Autodesk Fusion 360 part; units mm, degrees
note: some values were not read from the file. Chosen so that the rebuilt part matches the saved one: which face or edge a step refers to. Set by a fixed rule: which sketch regions a step uses; the direction of a hole.
(part 2 of 4)
sketch "Sketch67" plane through (0, 220, 0) normal (0, 1, 0) x (-1, 0, 0)
  line L0 (25, 0) -> (85, 0)
  line L1 (85, 0) -> (85, 30)
  line L2 (80, 25) -> (30, 25)
  line L3 (25, 30) -> (25, 0)
  line L4 (35, 26.3798) -> (35, 15.6202)
  line L5 (30.25, 21) -> (39.75, 21)
  line L6 (39.75, 21) -> (39.75, 17.5)
  line L7 (39.75, 17.5) -> (30.25, 17.5)
  line L8 (30.25, 17.5) -> (30.25, 21)
  line L9 (79.75, 21) -> (70.25, 21)
  line L10 (70.25, 21) -> (70.25, 17.5)
  line L11 (70.25, 17.5) -> (79.75, 17.5)
  line L12 (79.75, 17.5) -> (79.75, 21)
  line L13 (75, 25) -> (75, 17)
  line L14 (25, 25) -> (85, 25)
  line L15 (85, 30) -> (80, 30)
  line L16 (80, 30) -> (80, 25)
  line L17 (30, 25) -> (30, 30)
  line L18 (30, 30) -> (25, 30)
  dimension "d520" = 9.5
  dimension "d521" = 3.5
  dimension "d522" = 4
  dimension "d523" = 10
  dimension "d524" = 9.5
  dimension "d525" = 3.5
  dimension "d526" = 10
  dimension "d527" = 4
  constraint vertical L4
  constraint horizontal L5
  constraint vertical L6
  constraint horizontal L7
  constraint vertical L8
  constraint midpoint L4 L5
  constraint horizontal L9
  constraint vertical L10
  constraint horizontal L11
  constraint vertical L12
  constraint coincident L2 L13.start
  constraint perpendicular L2 L13
  constraint midpoint L9 L13
  measures "d520" distance of L5.start L5.end
  measures "d521" distance of L5.start L7.end
  measures "d522" distance of L2 L5
  measures "d523" distance of L3 L4
  measures "d524" distance of L9.start L9.end
  measures "d525" distance of L9.start L11.end
  measures "d526" distance of L1 L13
  measures "d527" distance of L9 L14
extrude "Extrude94" cut sketch "Sketch67" against normal blind 8 contours L4 L5 L6 L7 | L4 L5 L7 L8 | L9 L11 L12 L13 | L9 L10 L11 L13 bodies 3
sketch "Sketch68" plane through (0, 0, 25) normal (0, 0, 1) x (-1, 0, 0)
  line L0 (-25, -115) -> (-25, -75)
  line L1 (-25, -75) -> (-85, -75)
  line L2 (-85, -75) -> (-85, -115)
  line L3 (-85, -115) -> (-25, -115)
  line L4 (-85, -75) -> (-65, -75)
  line L5 (-65, -75) -> (-65, -115)
  line L6 (-65, -115) -> (-85, -115)
  line L7 (-85, -115) -> (-85, -75)
  constraint horizontal L4
  constraint vertical L5
  constraint horizontal L6
  constraint vertical L7
  constraint coincident L3 L5.end
  constraint coincident L1.end L2.start
sketch "Sketch70" plane through (85, 0, 0) normal (1, 0, 0) x (0, 1, 0)
  line L0 (115, 25) -> (115, 60)
  line L1 (115, 60) -> (75, 60)
  line L2 (75, 60) -> (75, 25)
  line L3 (75, 10) -> (115, 10)
  line L4 (75, 10) -> (75, 20)
  line L5 (115, 20) -> (75, 20)
  line L6 (115, 20) -> (115, 10)
  line L7 (75, 60) -> (115, 60)
  line L8 (115, 60) -> (115, 57)
  line L9 (115, 57) -> (75, 57)
  line L10 (75, 57) -> (75, 60)
  line L11 (75, 25) -> (115, 25)
  dimension "d537" = 40
  constraint coincident L0 L3.end
  constraint perpendicular L0 L3
  constraint coincident L2 L4.end
  constraint coincident L0 L5.start
  constraint perpendicular L4 L5
  constraint horizontal L7
  constraint vertical L8
  constraint horizontal L9
  constraint vertical L10
  constraint coincident L0 L8.end
  constraint coincident L1.end L2.start
  measures "d537" distance of L1 L5
sketch "Sketch71" plane through (0, 0, 57) normal (0, 0, -1) x (1, 0, 0)
  line L0 (85, -115) -> (93, -115)
  line L1 (93, -115) -> (93, -75)
  line L2 (93, -75) -> (85, -75)
  circle A0 centre (90.65, -110.5) radius 1.5
  line L3 (85, -115) -> (85, -75)
  circle A1 centre (90.65, -79.5) radius 1.5
  line L4 (85, -75) -> (85, -115)
  dimension "d543" = 3
  dimension "d544" = 5.65
  dimension "d545" = 3
  dimension "d546" = 5.65
  dimension "d547" = 31
  dimension "d548" = 4.5
  measures "d543" diameter of A0
  measures "d544" distance of A0.centre L3
  measures "d545" diameter of A1
  measures "d546" distance of L3 A1.centre
  measures "d547" distance of A0.centre A1.centre
  measures "d548" distance of L2 A1.centre
sketch "Sketch72" plane through (0, 0, 20) normal (0, 0, 1) x (-1, 0, 0)
  line L0 (-85, -75) -> (-95, -75)
  line L1 (-95, -75) -> (-95, -115)
  line L2 (-95, -115) -> (-85, -115)
  circle A0 centre (-106.15, -95) radius 9.5
  line L3 (-85, -75) -> (-85, -115)
  line L4 (-85, -115) -> (-85, -75)
  dimension "d552" = 19
  dimension "d553" = 21.15
  dimension "d554" = 20
  measures "d552" diameter of A0
  measures "d553" distance of A0.centre L3
  measures "d554" distance of L2 A0.centre
sketch "Sketch73" plane through (0, 115, 0) normal (0, 1, 0) x (-1, 0, 0)
  line L0 (-85, 60) -> (-93, 60)
  line L1 (-93, 60) -> (-93, 57)
  line L2 (-93, 57) -> (-85, 57)
  circle A0 centre (-55, 45) radius 10
  line L3 (-85, 57) -> (-85, 60)
sketch "Sketch74" plane through (0, 0, 90) normal (0, 0, 1) x (-1, 0, 0)
  circle A0 centre (-106.15, -95) radius 9.5
  circle A1 centre (-106.15, -95) radius 4
  dimension "d563" = 8
  constraint concentric A0 A1
  measures "d563" diameter of A1
sketch "Sketch76" plane through (0, 0, 60) normal (0, 0, 1) x (-1, 0, 0)
  circle A0 centre (-90.65, -110.5) radius 1.5
  circle A1 centre (-90.65, -79.5) radius 1.5
  line L0 (-93, -115) -> (-85, -115)
  line L1 (-85, -75) -> (-93, -75)
  line L2 (-93, -75) -> (-93, -115)
  line L3 (-80, -90) -> (-70, -90)
  line L4 (-70, -90) -> (-70, -100)
  line L5 (-70, -100) -> (-80, -100)
  line L6 (-80, -100) -> (-80, -90)
  line L7 (-85, -115) -> (-85, -75)
  dimension "d566" = 10
  dimension "d567" = 10
  constraint horizontal L3
  constraint vertical L4
  constraint horizontal L5
  constraint vertical L6
  measures "d566" distance of L3.start L3.end
  measures "d567" distance of L3.start L5.end
sketch "Sketch77" plane through (0, 0, 0) normal (0, 0, 1) x (1, 0, 0)
  line L0 (145, 120) -> (60, 120)
  line L1 (60, 120) -> (60, 150)
  line L2 (60, 150) -> (145, 150)
  line L3 (145, 150) -> (145, 120)
  dimension "d669" = 85
  constraint horizontal L0
  constraint vertical L1
  constraint horizontal L2
  constraint vertical L3
  measures "d669" distance of L1.end L2.end
sketch "Sketch78" plane through (0, 0, 10) normal (0, 0, 1) x (-1, 0, 0)
  line L0 (-145, -150) -> (-60, -150)
  line L1 (-60, -150) -> (-60, -120)
  line L2 (-60, -120) -> (-145, -120)
  line L3 (-145, -120) -> (-145, -150)
  circle A0 centre (-103.65, -135) radius 8.5
  line L4 (-77.5, -130) -> (-67.5, -130)
  line L5 (-67.5, -130) -> (-67.5, -140)
  line L6 (-67.5, -140) -> (-77.5, -140)
  line L7 (-77.5, -140) -> (-77.5, -130)
  circle A1 centre (-67.5, -130) radius 1.5
  circle A2 centre (-67.5, -140) radius 1.5
  circle A3 centre (-77.5, -140) radius 1.5
  circle A4 centre (-77.5, -130) radius 1.5
  circle A5 centre (-72.5, -135) radius 2.5
  line L8 (-139.8, -130) -> (-129.8, -130)
  line L9 (-129.8, -130) -> (-129.8, -140)
  line L10 (-129.8, -140) -> (-139.8, -140)
  line L11 (-139.8, -140) -> (-139.8, -130)
  line L12 (-145, -150) -> (-145, -120)
  line L13 (-60, -150) -> (-145, -150)
  circle A6 centre (-129.8, -130) radius 1.5
  circle A7 centre (-129.8, -140) radius 1.5
  circle A8 centre (-139.8, -130) radius 1.5
  circle A9 centre (-139.8, -140) radius 1.5
  circle A10 centre (-134.8, -135) radius 2.5
  dimension "d572" = 17
  dimension "d573" = 26.15
  dimension "d574" = 7.5
  dimension "d582" = 5
  dimension "d583" = 5
  dimension "d584" = 5
  dimension "d670" = 10
  dimension "d671" = 10
  dimension "d674" = 3
  dimension "d675" = 3
  dimension "d676" = 3
  dimension "d677" = 3
  dimension "d678" = 5
  dimension "d679" = 26.15
  dimension "d680" = 10
  dimension "d681" = 5
  constraint horizontal L4
  constraint vertical L5
  constraint horizontal L6
  constraint vertical L7
  constraint coincident L4.end L5.start
  constraint coincident L5.end L6.start
  constraint coincident L6.end L7.start
  constraint coincident L4.start L7.end
  constraint horizontal L8
  constraint vertical L9
  constraint horizontal L10
  constraint vertical L11
  constraint coincident L8.end L9.start
  constraint coincident L9.end L10.start
  constraint coincident L8.start L11.end
  constraint coincident L10.end L11.start
  measures "d572" diameter of A0
  measures "d573" distance of A0.centre L7
  measures "d574" distance of L1 L5
  measures "d582" distance of L4 A5.centre
  measures "d583" distance of L7 A5.centre
  measures "d584" diameter of A5
  measures "d670" distance of L8.start L8.end
  measures "d671" distance of L8.start L10.end
  measures "d674" diameter of A6
  measures "d675" diameter of A7
  measures "d676" diameter of A8
  measures "d677" diameter of A9
  measures "d678" diameter of A10
  measures "d679" distance of A0.centre L9
  measures "d680" distance of L5.end L6.end
  measures "d681" distance of L9 A10.centre
sketch "Sketch79" plane through (0, 0, 140) normal (0, 0, 1) x (-1, 0, 0)
  line L0 (-80, -100) -> (-70, -100)
  line L1 (-70, -100) -> (-70, -90)
  line L2 (-70, -90) -> (-80, -90)
  line L3 (-80, -90) -> (-80, -100)
  circle A0 centre (-75, -95) radius 2.5
  dimension "d587" = 5
  measures "d587" diameter of A0
sketch "Sketch80" plane through (0, 0, 0) normal (0, 0, 1) x (1, 0, 0)
  line L0 (120, 160) -> (25, 160)
  line L1 (25, 160) -> (25, 190)
  line L2 (25, 190) -> (120, 190)
  line L3 (120, 190) -> (120, 160)
  dimension "d593" = 95
  dimension "d594" = 30
  constraint horizontal L0
  constraint vertical L1
  constraint horizontal L2
  constraint vertical L3
  measures "d593" distance of L0.start L0.end
  measures "d594" distance of L0.start L2.end
sketch "Sketch81" plane through (0, 0, 90) normal (0, 0, 1) x (-1, 0, 0)
  circle A0 centre (-90.65, -110.5) radius 1.5
  circle A1 centre (-90.65, -79.5) radius 1.5
  line L0 (-93, -115) -> (-85, -115)
  line L1 (-85, -75) -> (-93, -75)
  line L2 (-93, -75) -> (-93, -115)
  line L3 (-93, -105) -> (-85, -105)
  line L4 (-85, -105) -> (-85, -115)
  line L5 (-85, -115) -> (-93, -115)
  line L6 (-93, -115) -> (-93, -105)
  line L7 (-93, -75) -> (-85, -75)
  line L8 (-85, -75) -> (-85, -85)
  line L9 (-85, -85) -> (-93, -85)
  line L10 (-93, -85) -> (-93, -75)
  line L11 (-85, -115) -> (-85, -75)
  constraint horizontal L3
  constraint vertical L4
  constraint horizontal L5
  constraint vertical L6
  constraint coincident L0 L4.end
  constraint coincident L2 L3.start
  constraint horizontal L7
  constraint vertical L8
  constraint horizontal L9
  constraint vertical L10
  constraint coincident L1.end L2.start
extrude "Extrude108" cut sketch "Sketch81" against normal blind 23 contours L0 L2 L3 L4 L5 L6 L11 | L1 L2 L7 L8 L9 L10 L11
sketch "Sketch82" plane through (0, 0, 15) normal (0, 0, 1) x (-1, 0, 0)
  line L0 (-120, -190) -> (-25, -190)
  line L1 (-25, -190) -> (-25, -160)
  line L2 (-25, -160) -> (-120, -160)
  line L3 (-120, -160) -> (-120, -190)
  circle A0 centre (-103.65, -175) radius 7.5
  line L4 (-77.5, -170) -> (-67.5, -170)
  line L5 (-67.5, -170) -> (-67.5, -180)
  line L6 (-67.5, -180) -> (-77.5, -180)
  line L7 (-77.5, -180) -> (-77.5, -170)
  circle A1 centre (-67.5, -170) radius 1.5
  circle A2 centre (-67.5, -180) radius 1.5
  circle A3 centre (-77.5, -180) radius 1.5
  circle A4 centre (-77.5, -170) radius 1.5
  line L8 (-57.5, -160) -> (-57.5, -190)
  line L9 (-47.5, -160) -> (-47.5, -190)
  dimension "d603" = 15
  dimension "d604" = 26.15
  dimension "d605" = 16.35
  dimension "d606" = 10
  dimension "d607" = 10
  constraint horizontal L4
  constraint vertical L5
  constraint horizontal L6
  constraint vertical L7
  constraint coincident L4.end L5.start
  constraint coincident L5.end L6.start
  constraint coincident L6.end L7.start
  constraint coincident L4.start L7.end
  constraint coincident L2 L8.start
  constraint coincident L0 L8.end
  constraint perpendicular L0 L8
  constraint coincident L2 L9.start
  constraint coincident L0 L9.end
  constraint perpendicular L0 L9
  measures "d603" diameter of A0
  measures "d604" distance of A0.centre L7
  measures "d605" distance of L3 A0.centre
  measures "d606" distance of L5 L8
  measures "d607" distance of L8 L9
sketch "Sketch89" plane through (0, 190, 0) normal (0, 1, 0) x (-1, 0, 0)
  line L0 (-47.5, 15) -> (-47.5, 65)
  line L1 (-47.5, 65) -> (-57.5, 65)
  line L2 (-57.5, 65) -> (-57.5, 15)
  circle A0 centre (-47.5, 55) radius 10
  line L3 (-57.5, 15) -> (-47.5, 15)
  dimension "d623" = 20
  constraint tangent L1 A0
  constraint tangent L2 A0
  measures "d623" diameter of A0
sketch "Sketch90" plane through (0, 0, 65) normal (0, 0, 1) x (-1, 0, 0)
  line L0 (-57.5, -160) -> (-57.5, -190)
  line L1 (-57.5, -190) -> (-47.5, -190)
  line L2 (-47.5, -190) -> (-47.5, -160)
  line L3 (-47.5, -160) -> (-57.5, -160)
  line L4 (-47.5, -190) -> (-47.5, -198)
  line L5 (-47.5, -160) -> (-40, -160)
  line L6 (-40, -160) -> (-40, -198)
  line L7 (-40, -198) -> (-47.5, -198)
  line L8 (-47.5, -198) -> (-47.5, -160)
  line L9 (-40, -198) -> (-150, -198)
  line L10 (-150, -198) -> (-150, -228)
  line L11 (-150, -228) -> (-40, -228)
  line L12 (-40, -228) -> (-40, -198)
  circle A0 centre (-47.5, -198) radius 1.5
  circle A1 centre (-68, -223) radius 1.5
  circle A2 centre (-140, -223) radius 1.5
  line L13 (-150, -228) -> (-40, -228)
  point P0 (-47.5, -190)
  dimension "d643" = 8
  dimension "d644" = 110
  dimension "d645" = 30
  dimension "d652" = 3
  dimension "d655" = 3
  dimension "d656" = 3
  dimension "d657" = 25
  dimension "d658" = 25
  dimension "d659" = 72
  dimension "d660" = 28
  dimension "d733" = 8
  constraint coincident P0 L1.end
  constraint perpendicular L1 L4
  constraint horizontal L5
  constraint vertical L6
  constraint horizontal L7
  constraint vertical L8
  constraint coincident L2.end L3.start
  constraint horizontal L9
  constraint vertical L10
  constraint horizontal L11
  constraint vertical L12
  constraint coincident L4.end L7.end
  constraint horizontal L13
  measures "d643" distance of P0 L4.end
  measures "d644" distance of L6.end L9.end
  measures "d645" distance of L6.end L11.end
  measures "d652" diameter of A0
  measures "d655" diameter of A1
  measures "d656" diameter of A2
  measures "d657" distance of L9 A1.centre
  measures "d658" distance of L9 A2.centre
  measures "d659" distance of A1.centre A2.centre
  measures "d660" distance of L12 A1.centre
  measures "d733" distance of L9 P0
sketch "Sketch92" plane through (0, 0, 0) normal (0, 0, 1) x (1, 0, 0)
sketch "Sketch93" plane through (0, 0, 0) normal (0, 0, 1) x (1, 0, 0)
  line L0 (160.9039, 76.8073) -> (132.9039, 76.8073)
  line L1 (132.9039, 76.8073) -> (132.9039, 116.8073)
  line L2 (132.9039, 116.8073) -> (160.9039, 116.8073)
  line L3 (160.9039, 116.8073) -> (160.9039, 76.8073)
  line L4 (160.9039, 76.8073) -> (152.9039, 76.8073)
  line L5 (152.9039, 76.8073) -> (152.9039, 86.8073)
  line L6 (152.9039, 86.8073) -> (160.9039, 86.8073)
  line L7 (160.9039, 86.8073) -> (160.9039, 76.8073)
  line L8 (160.9039, 116.8073) -> (152.9039, 116.8073)
  line L9 (152.9039, 116.8073) -> (152.9039, 106.8073)
  line L10 (152.9039, 106.8073) -> (160.9039, 106.8073)
  line L11 (160.9039, 106.8073) -> (160.9039, 116.8073)
  line L12 (147.9039, 91.8073) -> (137.9039, 91.8073)
  line L13 (137.9039, 91.8073) -> (137.9039, 101.8073)
  line L14 (137.9039, 101.8073) -> (147.9039, 101.8073)
  line L15 (147.9039, 101.8073) -> (147.9039, 91.8073)
  circle A0 centre (158.5539, 112.3073) radius 1.5
  circle A1 centre (158.5539, 81.3073) radius 1.5
  line L16 (152.9039, 106.8073) -> (152.9039, 86.8073)
  dimension "d686" = 28
  dimension "d687" = 40
  dimension "d688" = 8
  dimension "d689" = 10
  dimension "d690" = 8
  dimension "d691" = 10
  dimension "d692" = 10
  dimension "d693" = 10
  dimension "d694" = 15
  dimension "d695" = 5
  dimension "d700" = 3
  dimension "d701" = 3
  dimension "d702" = 2.35
  dimension "d703" = 4.5
  dimension "d704" = 2.35
  dimension "d705" = 4.5
  constraint horizontal L0
  constraint vertical L1
  constraint horizontal L2
  constraint vertical L3
  constraint horizontal L4
  constraint vertical L5
  constraint horizontal L6
  constraint vertical L7
  constraint horizontal L8
  constraint vertical L9
  constraint horizontal L10
  constraint vertical L11
  constraint horizontal L12
  constraint vertical L13
  constraint horizontal L14
  constraint vertical L15
  measures "d686" distance of L0.start L0.end
  measures "d687" distance of L0.start L2.end
  measures "d688" distance of L0.start L4.end
  measures "d689" distance of L0.start L6.end
  measures "d690" distance of L2.end L8.end
  measures "d691" distance of L2.end L10.end
  measures "d692" distance of L12.start L12.end
  measures "d693" distance of L12.start L14.end
  measures "d694" distance of L2 L14
  measures "d695" distance of L1 L13
  measures "d700" diameter of A0
  measures "d701" diameter of A1
  measures "d702" distance of L11 A0.centre
  measures "d703" distance of L8 A0.centre
  measures "d704" distance of L3 A1.centre
  measures "d705" distance of L4 A1.centre
sketch "Sketch94" plane through (152.9039, 0, 0) normal (1, 0, 0) x (0, 1, 0)
  line L0 (76.8073, 0) -> (76.8073, -47)
  line L1 (76.8073, -47) -> (116.8073, -47)
  line L2 (116.8073, -47) -> (116.8073, 0)
  line L3 (76.8073, -47) -> (116.8073, -47)
  line L4 (116.8073, -47) -> (116.8073, -38)
  line L5 (116.8073, -38) -> (76.8073, -38)
  line L6 (76.8073, -38) -> (76.8073, -47)
  line L7 (116.8073, 0) -> (76.8073, 0)
  dimension "d712" = 9
  constraint horizontal L3
  constraint vertical L4
  constraint horizontal L5
  constraint vertical L6
  constraint coincident L2 L4.end
  constraint coincident L0.end L1.start
  measures "d712" distance of L0.end L5.end
sketch "Sketch95" plane through (0, 0, 15) normal (0, 0, 1) x (-1, 0, 0)
  line L0 (-120, -160) -> (-147.5, -160)
  line L1 (-147.5, -160) -> (-147.5, -190)
  line L2 (-147.5, -190) -> (-120, -190)
  line L3 (-129.8, -180) -> (-139.8, -180)
  line L4 (-139.8, -180) -> (-139.8, -170)
  line L5 (-139.8, -170) -> (-129.8, -170)
  line L6 (-129.8, -170) -> (-129.8, -180)
  circle A0 centre (-139.8, -180) radius 1.5
  circle A1 centre (-139.8, -170) radius 1.5
  circle A2 centre (-129.8, -170) radius 1.5
  circle A3 centre (-129.8, -180) radius 1.5
  line L7 (-120, -190) -> (-120, -160)
  point P0 (-103.65, -175)
  dimension "d717" = 10
  dimension "d718" = 10
  dimension "d719" = 26.15
  dimension "d720" = 10
  dimension "d721" = 3
  dimension "d722" = 3
  dimension "d723" = 3
  dimension "d724" = 3
  constraint horizontal L3
  constraint vertical L4
  constraint horizontal L5
  constraint vertical L6
  constraint coincident L3.end L4.start
  constraint coincident L4.end L5.start
  constraint coincident L5.end L6.start
  constraint coincident L3.start L6.end
  measures "d717" distance of L3.start L3.end
  measures "d718" distance of L3.start L5.end
  measures "d719" distance of L6 P0
  measures "d720" distance of L0 L5
  measures "d721" diameter of A0
  measures "d722" diameter of A1
  measures "d723" diameter of A2
  measures "d724" diameter of A3
sketch "Sketch96" plane through (0, 0, 83) normal (0, 0, 1) x (-1, 0, 0)
  line L0 (-147.9039, -101.8073) -> (-137.9039, -101.8073)
  line L1 (-137.9039, -101.8073) -> (-137.9039, -91.8073)
  line L2 (-137.9039, -91.8073) -> (-147.9039, -91.8073)
  line L3 (-147.9039, -91.8073) -> (-147.9039, -101.8073)
  circle A0 centre (-142.9039, -96.8073) radius 2.5
  dimension "d727" = 5
  measures "d727" diameter of A0
sketch "Sketch97" plane through (0, 0, 15) normal (0, 0, 1) x (-1, 0, 0)
  line L0 (-149.8, -190) -> (-149.8, -160)
  line L1 (-139.8, -180) -> (-139.8, -170)
  line L2 (-147.5, -190) -> (-149.8, -190)
  line L3 (-149.8, -160) -> (-147.5, -160)
  line L4 (-149.8, -190) -> (-159.8, -190)
  line L5 (-159.8, -190) -> (-159.8, -160)
  line L6 (-159.8, -160) -> (-149.8, -160)
  line L7 (-149.8, -160) -> (-149.8, -190)
  line L8 (-147.5, -190) -> (-147.5, -160)
  dimension "d734" = 10
  dimension "d735" = 10
  constraint vertical L0
  constraint perpendicular L0 L2
  constraint perpendicular L0 L3
  constraint horizontal L4
  constraint vertical L5
  constraint horizontal L6
  constraint vertical L7
  constraint perpendicular L3 L8
  measures "d734" distance of L0 L1
  measures "d735" distance of L0.start L4.end
sketch "Sketch98" plane through (0, 0, 15) normal (0, 0, 1) x (-1, 0, 0)
sketch "Sketch99" plane through (0, 190, 0) normal (0, 1, 0) x (-1, 0, 0)
  line L0 (-149.8, 15) -> (-149.8, 65)
  line L1 (-149.8, 65) -> (-159.8, 65)
  line L2 (-159.8, 65) -> (-159.8, 15)
  circle A0 centre (-159.8, 55) radius 10
  line L3 (-159.8, 55) -> (-169.8, 55)
  line L4 (-159.8, 55) -> (-167.3, 55)
  line L5 (-167.3, 55) -> (-167.3, 65)
  line L6 (-167.3, 65) -> (-159.8, 65)
  line L7 (-159.8, 65) -> (-159.8, 55)
  line L8 (-159.8, 15) -> (-149.8, 15)
  dimension "d740" = 20
  dimension "d741" = 7.5
  constraint coincident L2 A0.centre
  constraint tangent L1 A0
  constraint coincident A0.centre L3.start
  constraint coincident A0 L3.end
  constraint perpendicular L2 L3
  constraint horizontal L4
  constraint vertical L5
  constraint horizontal L6
  constraint vertical L7
  measures "d740" diameter of A0
  measures "d741" distance of A0.centre L4.end
sketch "Sketch100" plane through (0, 0, 0) normal (0, 0, 1) x (1, 0, 0)
  line L0 (50, 0) -> (110, 0)
  line L1 (110, 0) -> (110, -45)
  line L2 (110, -45) -> (50, -45)
  line L3 (50, -45) -> (50, 0)
  dimension "d752" = 60
  dimension "d753" = 45
  constraint horizontal L0
  constraint vertical L1
  constraint horizontal L2
  constraint vertical L3
  measures "d752" distance of L0.start L0.end
  measures "d753" distance of L0.start L2.end
extrude "Extrude139" add sketch "Sketch100" along normal blind 30 separate body makes body 5
sketch "Sketch101" plane through (0, -45, 0) normal (0, -1, 0) x (1, 0, 0)
  line L0 (50, 0) -> (110, 0)
  line L1 (110, 0) -> (110, 30)
  line L2 (110, 30) -> (50, 30)
  line L3 (50, 30) -> (50, 0)
  line L4 (55, 5) -> (60, 5)
  line L5 (60, 5) -> (60, 0)
  line L6 (60, 0) -> (55, 0)
  line L7 (55, 0) -> (55, 5)
  line L8 (100, 5) -> (105, 5)
  line L9 (105, 5) -> (105, 0)
  line L10 (105, 0) -> (100, 0)
  line L11 (100, 0) -> (100, 5)
  line L12 (55, 5) -> (54, 5)
  line L13 (54, 5) -> (55, 0)
  line L14 (60, 5) -> (61, 5)
  line L15 (60, 0) -> (61, 5)
  line L16 (100, 5) -> (99, 5)
  line L17 (99, 5) -> (100, 0)
  line L18 (105, 5) -> (106, 5)
  line L19 (106, 5) -> (105, 0)
  line L20 (80, 0) -> (80, 12.75)
  circle A0 centre (80, 12.75) radius 7.5
  circle A1 centre (54, 5) radius 1
  circle A2 centre (61, 5) radius 1
  circle A3 centre (60, 0) radius 1
  circle A4 centre (55, 0) radius 1
  circle A5 centre (99, 5) radius 1
  circle A6 centre (106, 5) radius 1
  circle A7 centre (105, 0) radius 1
  circle A8 centre (100, 0) radius 1
  dimension "d756" = 1
  dimension "d757" = 1
  dimension "d758" = 1
  dimension "d759" = 1
  dimension "d760" = 12.75
  dimension "d761" = 15
  dimension "d762" = 2
  dimension "d763" = 2
  dimension "d764" = 2
  dimension "d765" = 2
  dimension "d766" = 2
  dimension "d767" = 2
  dimension "d768" = 2
  dimension "d769" = 2
  constraint horizontal L4
  constraint vertical L5
  constraint horizontal L6
  constraint vertical L7
  constraint coincident L0 L5.end
  constraint horizontal L8
  constraint vertical L9
  constraint horizontal L10
  constraint vertical L11
  constraint coincident L0 L9.end
  constraint perpendicular L7 L12
  constraint perpendicular L7 L14
  constraint perpendicular L11 L16
  constraint perpendicular L9 L18
  constraint midpoint L0 L20.start
  constraint perpendicular L0 L20
  constraint coincident L20.end A0.centre
  constraint coincident L12.end L13.start
  constraint coincident L14.end L15.end
  constraint coincident L5.end L6.start
  constraint coincident L6.end L7.start
  constraint coincident L16.end L17.start
  constraint coincident L18.end L19.start
  constraint coincident L9.end L10.start
  constraint coincident L10.end L11.start
  measures "d756" distance of L4.start L12.end
  measures "d757" distance of L4.end L14.end
  measures "d758" distance of L8.start L16.end
  measures "d759" distance of L8.end L18.end
  measures "d760" distance of L20.start L20.end
  measures "d761" diameter of A0
  measures "d762" diameter of A1
  measures "d763" diameter of A2
  measures "d764" diameter of A3
  measures "d765" diameter of A4
  measures "d766" diameter of A5
  measures "d767" diameter of A6
  measures "d768" diameter of A7
  measures "d769" diameter of A8
extrude "Extrude140" cut sketch "Sketch101" against normal blind 45 contours L0 L6 L7 A4 | L7 L13 A4 | L0 L13 A4 | L0 L4 L5 L6 L7 A3 A4 | L7 L13 A1 A4 | L0 L5 L6 A3 | L12 L13 A1 | L12 L13 A1 | L0 L15 A3 | L5 L15 A3 | L5 L15 A2 A3 | L14 L15 A2 | L14 L15 A2 | L0 L17 A8 | L0 L10 L11 A8 | L11 L17 A8 | L11 L17 A5 A8 | L0 L8 L9 L10 L11 A7 A8 | L0 L19 A7 | L16 L17 A5 | L16 L17 A5 | L0 L9 L10 A7 | L9 L19 A7 | L9 L19 A6 A7 | L18 L19 A6 | L18 L19 A6 bodies 5
hole "Hole30" at (80, -45, 12.75) direction (0, 1, 0) diameter 13.9 depth 15 tip angle 180 countersink diameter 15 countersink angle 30 bodies 5
sketch "Sketch102" plane through (0, 0, 0) normal (0, 1, 0) x (-1, 0, 0)
  arc A0 (-60.1961, 0.9806) -> (-61, 0) centre (-60, 0) ccw
  line L0 (-60.1961, 0.9806) -> (-60.8039, 4.0194)
  arc A1 (-60, 5) -> (-60.8039, 4.0194) centre (-61, 5) ccw
  line L1 (-60, 5) -> (-55, 5)
  arc A2 (-54.1961, 4.0194) -> (-55, 5) centre (-54, 5) ccw
  line L2 (-54.1961, 4.0194) -> (-54.8039, 0.9806)
  arc A3 (-54, 0) -> (-54.8039, 0.9806) centre (-55, 0) ccw
  line L3 (-54, 0) -> (-50, 0)
  line L4 (-50, 0) -> (-50, 30)
  line L5 (-50, 30) -> (-110, 30)
  line L6 (-110, 30) -> (-110, 0)
  line L7 (-110, 0) -> (-106, 0)
  arc A4 (-105.1961, 0.9806) -> (-106, 0) centre (-105, 0) ccw
  line L8 (-105.1961, 0.9806) -> (-105.8039, 4.0194)
  arc A5 (-105, 5) -> (-105.8039, 4.0194) centre (-106, 5) ccw
  line L9 (-105, 5) -> (-100, 5)
  arc A6 (-99.1961, 4.0194) -> (-100, 5) centre (-99, 5) ccw
  line L10 (-99.1961, 4.0194) -> (-99.8039, 0.9806)
  arc A7 (-99, 0) -> (-99.8039, 0.9806) centre (-100, 0) ccw
  line L11 (-99, 0) -> (-61, 0)
  line L12 (-80, 0) -> (-80, 12.75)
  circle A8 centre (-80, 12.75) radius 11.5
  dimension "d777" = 12.75
  dimension "d778" = 23
  constraint midpoint L11 L12.start
  constraint perpendicular L11 L12
  constraint coincident L12.end A8.centre
  measures "d777" distance of L12.start L12.end
  measures "d778" diameter of A8
hole "Hole31" at (80, 0, 12.75) direction (0, -1, 0) diameter 21 depth 30 tip angle 180 counterbore diameter 23 counterbore depth 3 bodies 5
sketch "Sketch103" plane through (0, 0, 30) normal (0, 0, 1) x (-1, 0, 0)
  line L0 (-50, 45) -> (-110, 45)
  line L1 (-110, 45) -> (-110, 0)
  line L2 (-110, 0) -> (-50, 0)
  line L3 (-50, 0) -> (-50, 45)
  line L4 (-90, 0) -> (-110, 0)
  line L5 (-110, 0) -> (-110, 45)
  line L6 (-110, 45) -> (-90, 45)
  line L7 (-90, 45) -> (-90, 0)
  constraint horizontal L4
  constraint vertical L5
  constraint horizontal L6
  constraint vertical L7
  constraint coincident L0.end L1.start
  constraint coincident L2 L4.start
extrude "Extrude141" add sketch "Sketch103" along normal blind 60 contours L0 L1 L2 L4 L5 L6 L7 bodies 5
sketch "Sketch104" plane through (0, -45, 0) normal (0, -1, 0) x (1, 0, 0)
  circle A0 centre (80, 12.75) radius 7.5
  arc A1 (61, 0) -> (60.1961, 0.9806) centre (60, 0) ccw
  line L0 (61, 0) -> (99, 0)
  arc A2 (99.8039, 0.9806) -> (99, 0) centre (100, 0) ccw
  line L1 (99.8039, 0.9806) -> (99.1961, 4.0194)
  arc A3 (100, 5) -> (99.1961, 4.0194) centre (99, 5) ccw
  line L2 (100, 5) -> (105, 5)
  arc A4 (105.8039, 4.0194) -> (105, 5) centre (106, 5) ccw
  line L3 (105.8039, 4.0194) -> (105.1961, 0.9806)
  arc A5 (106, 0) -> (105.1961, 0.9806) centre (105, 0) ccw
  line L4 (106, 0) -> (110, 0)
  line L5 (110, 0) -> (110, 90)
  line L6 (110, 90) -> (90, 90)
  line L7 (90, 90) -> (90, 30)
  line L8 (90, 30) -> (50, 30)
  line L9 (50, 30) -> (50, 0)
  line L10 (50, 0) -> (54, 0)
  arc A6 (54.8039, 0.9806) -> (54, 0) centre (55, 0) ccw
  line L11 (54.8039, 0.9806) -> (54.1961, 4.0194)
  arc A7 (55, 5) -> (54.1961, 4.0194) centre (54, 5) ccw
  line L12 (55, 5) -> (60, 5)
  arc A8 (60.8039, 4.0194) -> (60, 5) centre (61, 5) ccw
  line L13 (60.8039, 4.0194) -> (60.1961, 0.9806)
  circle A9 centre (80, 40) radius 10
  constraint tangent L7 A9
extrude "Extrude142" add sketch "Sketch104" against normal blind 45 contours L7 L8 A9 bodies 5
sketch "Sketch105" plane through (110, 0, 0) normal (1, 0, 0) x (0, 1, 0)
  line L0 (-45, 0) -> (0, 0)
  line L1 (0, 0) -> (0, 90)
  line L2 (0, 90) -> (-45, 90)
  line L3 (-45, 90) -> (-45, 0)
  line L4 (-45, 90) -> (0, 90)
  line L5 (0, 90) -> (0, 57)
  line L6 (0, 57) -> (-45, 57)
  line L7 (-45, 57) -> (-45, 90)
  line L8 (-45, 90) -> (-32.5, 90)
  line L9 (-32.5, 90) -> (-32.5, 57)
  line L10 (-32.5, 57) -> (-45, 57)
  line L11 (-45, 57) -> (-45, 90)
  line L12 (0, 90) -> (-12.5, 90)
  line L13 (-12.5, 90) -> (-12.5, 57)
  line L14 (-12.5, 57) -> (0, 57)
  line L15 (0, 57) -> (0, 90)
  line L16 (-45, 57) -> (0, 57)
  line L17 (0, 57) -> (0, 67)
  line L18 (0, 67) -> (-45, 67)
  line L19 (-45, 67) -> (-45, 57)
  line L20 (-45, 0) -> (0, 0)
  line L21 (0, 0) -> (0, 10)
  line L22 (0, 10) -> (-45, 10)
  line L23 (-45, 10) -> (-45, 0)
  line L24 (-45, 10) -> (0, 10)
  line L25 (0, 10) -> (0, 20)
  line L26 (0, 20) -> (-45, 20)
  line L27 (-45, 20) -> (-45, 10)
  dimension "d788" = 33
  dimension "d789" = 12.5
  dimension "d790" = 12.5
  dimension "d791" = 10
  dimension "d792" = 10
  dimension "d793" = 10
  constraint horizontal L4
  constraint vertical L5
  constraint horizontal L6
  constraint vertical L7
  constraint coincident L2.end L3.start
  constraint horizontal L8
  constraint vertical L9
  constraint horizontal L10
  constraint vertical L11
  constraint horizontal L12
  constraint vertical L13
  constraint horizontal L14
  constraint vertical L15
  constraint coincident L1.end L2.start
  constraint horizontal L16
  constraint vertical L17
  constraint horizontal L18
  constraint vertical L19
  constraint coincident L15 L17.end
  constraint horizontal L20
  constraint vertical L21
  constraint horizontal L22
  constraint vertical L23
  constraint coincident L1 L21.end
  constraint coincident L0.start L3.end
  constraint horizontal L24
  constraint vertical L25
  constraint horizontal L26
  constraint vertical L27
  constraint coincident L1 L25.end
  measures "d788" distance of L2.end L6.end
  measures "d789" distance of L2.end L8.end
  measures "d790" distance of L1.end L12.end
  measures "d791" distance of L6.end L18.end
  measures "d792" distance of L0.start L22.end
  measures "d793" distance of L22.end L26.end
extrude "Extrude143" add sketch "Sketch105" along normal blind 8 contours L1 L3 L22 L24 L25 L26 L27 | L3 L6 L7 L9 L10 L11 L16 L18 L19 | L1 L5 L6 L13 L14 L15 L16 L17 L18 | L6 L9 L13 L16 L18 | L2 L4 L9 L13 L18 bodies 5
sketch "Sketch106" plane through (0, 0, 67) normal (0, 0, 1) x (-1, 0, 0)
  line L0 (-110, 32.5) -> (-110, 45)
  line L1 (-110, 45) -> (-118, 45)
  line L2 (-118, 45) -> (-118, 32.5)
  line L3 (-118, 32.5) -> (-110, 32.5)
  circle A0 centre (-115.65, 38) radius 1.5
  dimension "d796" = 3
  dimension "d797" = 5.5
  dimension "d798" = 2.35
  measures "d796" diameter of A0
  measures "d797" distance of L3 A0.centre
  measures "d798" distance of L2 A0.centre
sketch "Sketch107" plane through (0, 0, 67) normal (0, 0, 1) x (-1, 0, 0)
  line L0 (-110, 0) -> (-110, 12.5)
  line L1 (-110, 12.5) -> (-118, 12.5)
  line L2 (-118, 12.5) -> (-118, 0)
  line L3 (-118, 0) -> (-110, 0)
  circle A0 centre (-115.65, 7) radius 1.5
  dimension "d799" = 3
  dimension "d800" = 5.5
  dimension "d801" = 2.35
  measures "d799" diameter of A0
  measures "d800" distance of L1 A0.centre
  measures "d801" distance of L2 A0.centre
sketch "Sketch108" plane through (0, 0, 90) normal (0, 0, 1) x (-1, 0, 0)
  line L0 (-90, 45) -> (-110, 45)
  line L1 (-110, 45) -> (-110, 32.5)
  line L2 (-110, 32.5) -> (-118, 32.5)
  line L3 (-118, 32.5) -> (-118, 12.5)
  line L4 (-118, 12.5) -> (-110, 12.5)
  line L5 (-110, 12.5) -> (-110, 0)
  line L6 (-110, 0) -> (-90, 0)
  line L7 (-90, 0) -> (-90, 45)
  line L8 (-90, 0) -> (-100, 0)
  line L9 (-100, 0) -> (-100, 10)
  line L10 (-100, 10) -> (-90, 10)
  line L11 (-90, 10) -> (-90, 0)
  line L12 (-90, 45) -> (-100, 45)
  line L13 (-100, 45) -> (-100, 35)
  line L14 (-100, 35) -> (-90, 35)
  line L15 (-90, 35) -> (-90, 45)
  circle A0 centre (-100, 10) radius 1
  circle A1 centre (-100, 0) radius 1
  circle A2 centre (-90, 10) radius 1
  circle A3 centre (-100, 35) radius 1
  circle A4 centre (-100, 45) radius 1
  circle A5 centre (-90, 35) radius 1
  circle A6 centre (-95, 5) radius 2.5
  circle A7 centre (-95, 40) radius 2.5
  dimension "d808" = 2
  dimension "d809" = 2
  dimension "d810" = 2
  dimension "d811" = 2
  dimension "d812" = 2
  dimension "d813" = 2
  dimension "d814" = 5
  dimension "d815" = 5
  constraint horizontal L8
  constraint vertical L9
  constraint horizontal L10
  constraint vertical L11
  constraint coincident L6.end L7.start
  constraint horizontal L12
  constraint vertical L13
  constraint horizontal L14
  constraint vertical L15
  constraint coincident L0.start L7.end
  constraint coincident L9.end L10.start
  constraint coincident L8.end L9.start
  constraint coincident L10.end L11.start
  constraint coincident L13.end L14.start
  constraint coincident L12.end L13.start
  constraint coincident L14.end L15.start
  measures "d808" diameter of A0
  measures "d809" diameter of A1
  measures "d810" diameter of A2
  measures "d811" diameter of A3
  measures "d812" diameter of A4
  measures "d813" diameter of A5
  measures "d814" diameter of A6
  measures "d815" diameter of A7
extrude "Extrude144" cut sketch "Sketch108" against normal blind 27.5 contours A6 | A7 bodies 5
extrude "Extrude145" cut sketch "Sketch108" against normal blind 5 contours L0 L7 L12 L13 L14 L15 A3 A4 A5 | L0 L12 L13 A4 | L7 L14 L15 A5 | L0 L13 A4 | L7 L14 A5 | L13 L14 A3 | L13 L14 A3 | L7 L10 A2 | L7 L10 L11 A2 | L6 L7 L8 L9 L10 L11 A0 A1 A2 | L9 L10 A0 | L9 L10 A0 | L6 L8 L9 A1 | L6 L9 A1 bodies 5
extrude "Extrude146" cut sketch "Sketch107" sketch "Sketch106" against normal blind 10 contours A0 of sketch 2 contours A0 bodies 5
sketch "Sketch109" plane through (90, 0, 0) normal (-1, 0, 0) x (0, -1, 0)
  line L0 (11, 90) -> (11, 85)
  line L1 (11, 85) -> (0, 85)
  line L2 (0, 85) -> (0, 40)
  line L3 (0, 40) -> (45, 40)
  line L4 (45, 40) -> (45, 85)
  line L5 (45, 85) -> (34, 85)
  line L6 (34, 85) -> (34, 90)
  line L7 (34, 90) -> (11, 90)
  line L8 (0, 79) -> (10, 79)
  line L9 (10, 79) -> (10, 76)
  line L10 (10, 76) -> (0, 76)
  line L11 (0, 76) -> (0, 79)
  line L12 (45, 76) -> (35, 76)
  line L13 (35, 76) -> (35, 79)
  line L14 (35, 79) -> (45, 79)
  line L15 (45, 79) -> (45, 76)
  dimension "d822" = 10
  dimension "d823" = 3
  dimension "d824" = 6
  dimension "d825" = 10
  dimension "d826" = 3
  dimension "d827" = 6
  constraint horizontal L8
  constraint vertical L9
  constraint horizontal L10
  constraint vertical L11
  constraint coincident L2 L8.start
  constraint horizontal L12
  constraint vertical L13
  constraint horizontal L14
  constraint vertical L15
  constraint coincident L4 L12.start
  measures "d822" distance of L8.start L8.end
  measures "d823" distance of L8.start L10.end
  measures "d824" distance of L1 L8
  measures "d825" distance of L12.start L12.end
  measures "d826" distance of L12.start L14.end
  measures "d827" distance of L5 L14
extrude "Extrude147" cut sketch "Sketch109" against normal blind 10 contours L2 L8 L9 L10 L11 | L4 L12 L13 L14 L15 bodies 5
sketch "Sketch110" plane through (0, 0, 0) normal (0, 0, 1) x (1, 0, 0)
  line L0 (150, 0) -> (170, 0)
  line L1 (170, 0) -> (170, -45)
  line L2 (170, -45) -> (150, -45)
  line L3 (150, -45) -> (150, 0)
  line L4 (170, 0) -> (180, 0)
  line L5 (180, 0) -> (180, -45)
  line L6 (180, -45) -> (170, -45)
  line L7 (170, -45) -> (170, 0)
  dimension "d830" = 20
  dimension "d831" = 45
  dimension "d832" = 45
  constraint horizontal L0
  constraint vertical L1
  constraint horizontal L2
  constraint vertical L3
  constraint horizontal L4
  constraint vertical L5
  constraint horizontal L6
  constraint vertical L7
  measures "d830" distance of L0.start L0.end
  measures "d831" distance of L0.start L2.end
  measures "d832" distance of L0.end L1.end
extrude "Extrude148" add sketch "Sketch110" along normal blind 80 separate body contours L0 L1 L2 L3 L7 makes body 6
extrude "Extrude149" add sketch "Sketch110" along normal blind 10 contours L1 L4 L5 L6 L7 bodies 6
sketch "Sketch111" plane through (170, 0, 0) normal (1, 0, 0) x (0, 1, 0)
  line L0 (-45, 10) -> (0, 10)
  line L1 (0, 10) -> (0, 80)
  line L2 (0, 80) -> (-45, 80)
  line L3 (-45, 80) -> (-45, 10)
  line L4 (-45, 80) -> (0, 80)
  line L5 (0, 80) -> (0, 47)
  line L6 (0, 47) -> (-45, 47)
  line L7 (-45, 47) -> (-45, 80)
  line L8 (-45, 47) -> (0, 47)
  line L9 (0, 47) -> (0, 57)
  line L10 (0, 57) -> (-45, 57)
  line L11 (-45, 57) -> (-45, 47)
  line L12 (-32.5, 80) -> (-12.5, 80)
  line L13 (-12.5, 80) -> (-12.5, 47)
  line L14 (-12.5, 47) -> (-32.5, 47)
  line L15 (-32.5, 47) -> (-32.5, 80)
  dimension "d838" = 33
  dimension "d839" = 45
  dimension "d840" = 10
  dimension "d841" = 20
  dimension "d842" = 12.5
  constraint horizontal L4
  constraint vertical L5
  constraint horizontal L6
  constraint vertical L7
  constraint coincident L2.end L3.start
  constraint horizontal L8
  constraint vertical L9
  constraint horizontal L10
  constraint vertical L11
  constraint horizontal L12
  constraint vertical L13
  constraint horizontal L14
  constraint vertical L15
  constraint coincident L6 L13.end
  constraint coincident L4 L12.start
  measures "d838" distance of L2.end L6.end
  measures "d839" distance of L6.end L5.end
  measures "d840" distance of L6.end L10.end
  measures "d841" distance of L12.start L12.end
  measures "d842" distance of L7 L15
extrude "Extrude150" add sketch "Sketch111" along normal blind 8 contours L3 L6 L7 L8 L10 L11 L15 | L1 L5 L6 L8 L9 L10 L13 | L6 L8 L10 L13 L14 L15 | L2 L4 L10 L12 L13 L15 bodies 6
sketch "Sketch112" plane through (0, 0, 57) normal (0, 0, 1) x (-1, 0, 0)
  line L0 (-170, 32.5) -> (-170, 45)
  line L1 (-170, 45) -> (-178, 45)
  line L2 (-178, 45) -> (-178, 32.5)
  line L3 (-178, 32.5) -> (-170, 32.5)
  circle A0 centre (-175.65, 38) radius 1.5
  line L4 (-180, 0) -> (-180, 45)
  dimension "d845" = 3
  dimension "d847" = 5.5
  dimension "d875" = 2.35
  measures "d845" diameter of A0
  measures "d847" distance of L3 A0.centre
  measures "d875" distance of L2 A0.centre
sketch "Sketch113" plane through (0, 0, 57) normal (0, 0, 1) x (-1, 0, 0)
  line L0 (-170, 0) -> (-170, 12.5)
  line L1 (-170, 12.5) -> (-178, 12.5)
  line L2 (-178, 12.5) -> (-178, 0)
  line L3 (-178, 0) -> (-170, 0)
  circle A0 centre (-175.65, 7) radius 1.5
  line L4 (-180, 0) -> (-180, 45)
  dimension "d848" = 3
  dimension "d849" = 5.5
  dimension "d876" = 2.35
  measures "d848" diameter of A0
  measures "d849" distance of L1 A0.centre
  measures "d876" distance of L2 A0.centre
extrude "Extrude151" cut sketch "Sketch113" sketch "Sketch112" against normal blind 10 contours A0 of sketch 2 contours A0 bodies 6
sketch "Sketch114" plane through (0, 0, 80) normal (0, 0, 1) x (-1, 0, 0)
  line L0 (-150, 45) -> (-170, 45)
  line L1 (-170, 45) -> (-170, 32.5)
  line L2 (-170, 32.5) -> (-178, 32.5)
  line L3 (-178, 32.5) -> (-178, 12.5)
  line L4 (-178, 12.5) -> (-170, 12.5)
  line L5 (-170, 12.5) -> (-170, 0)
  line L6 (-170, 0) -> (-150, 0)
  line L7 (-150, 0) -> (-150, 45)
  line L8 (-150, 0) -> (-160, 0)
  line L9 (-160, 0) -> (-160, 10)
  line L10 (-160, 10) -> (-150, 10)
  line L11 (-150, 10) -> (-150, 0)
  line L12 (-150, 45) -> (-160, 45)
  line L13 (-160, 45) -> (-160, 35)
  line L14 (-160, 35) -> (-150, 35)
  line L15 (-150, 35) -> (-150, 45)
  circle A0 centre (-160, 35) radius 1
  circle A1 centre (-160, 45) radius 1
  circle A2 centre (-150, 35) radius 1
  circle A3 centre (-160, 10) radius 1
  circle A4 centre (-160, 0) radius 1
  circle A5 centre (-150, 10) radius 1
  circle A6 centre (-155, 40) radius 2.5
  circle A7 centre (-155, 5) radius 2.5
  dimension "d853" = 2
  dimension "d854" = 2
  dimension "d855" = 2
  dimension "d856" = 2
  dimension "d857" = 2
  dimension "d858" = 2
  dimension "d859" = 5
  dimension "d860" = 5
  constraint horizontal L8
  constraint vertical L9
  constraint horizontal L10
  constraint vertical L11
  constraint coincident L6.end L7.start
  constraint horizontal L12
  constraint vertical L13
  constraint horizontal L14
  constraint vertical L15
  constraint coincident L0.start L7.end
  constraint coincident L13.end L14.start
  constraint coincident L12.end L13.start
  constraint coincident L14.end L15.start
  constraint coincident L9.end L10.start
  constraint coincident L8.end L9.start
  constraint coincident L10.end L11.start
  measures "d853" diameter of A0
  measures "d854" diameter of A1
  measures "d855" diameter of A2
  measures "d856" diameter of A3
  measures "d857" diameter of A4
  measures "d858" diameter of A5
  measures "d859" diameter of A6
  measures "d860" diameter of A7
extrude "Extrude152" cut sketch "Sketch114" against normal blind 27.5 contours A6 | A7 bodies 6
extrude "Extrude153" cut sketch "Sketch114" against normal blind 5 contours L0 L7 L12 L13 L14 L15 A0 A1 A2 | L0 L12 L13 A1 | L7 L14 L15 A2 | L0 L13 A1 | L7 L14 A2 | L13 L14 A0 | L13 L14 A0 | L7 L10 A5 | L7 L10 L11 A5 | L6 L7 L8 L9 L10 L11 A3 A4 A5 | L9 L10 A3 | L9 L10 A3 | L6 L8 L9 A4 | L6 L9 A4 bodies 6
sketch "Sketch115" plane through (150, 0, 0) normal (-1, 0, 0) x (0, -1, 0)
  line L0 (11, 80) -> (11, 75)
  line L1 (11, 75) -> (0, 75)
  line L2 (0, 75) -> (0, 0)
  line L3 (0, 0) -> (45, 0)
  line L4 (45, 0) -> (45, 75)
  line L5 (45, 75) -> (34, 75)
  line L6 (34, 75) -> (34, 80)
  line L7 (34, 80) -> (11, 80)
  line L8 (45, 66) -> (35, 66)
  line L9 (35, 66) -> (35, 69)
  line L10 (35, 69) -> (45, 69)
  line L11 (45, 69) -> (45, 66)
  line L12 (0, 66) -> (10, 66)
  line L13 (10, 66) -> (10, 69)
  line L14 (10, 69) -> (0, 69)
  line L15 (0, 69) -> (0, 66)
  dimension "d865" = 10
  dimension "d866" = 3
  dimension "d867" = 6
  dimension "d868" = 10
  dimension "d869" = 3
  dimension "d870" = 6
  constraint horizontal L8
  constraint vertical L9
  constraint horizontal L10
  constraint vertical L11
  constraint coincident L4 L8.start
  constraint horizontal L12
  constraint vertical L13
  constraint horizontal L14
  constraint vertical L15
  constraint coincident L2 L12.start
  measures "d865" distance of L8.start L8.end
  measures "d866" distance of L8.start L10.end
  measures "d867" distance of L5 L10
  measures "d868" distance of L12.start L12.end
  measures "d869" distance of L12.start L14.end
  measures "d870" distance of L1 L14
extrude "Extrude154" cut sketch "Sketch115" against normal blind 10 contours L2 L12 L13 L14 L15 | L4 L8 L9 L10 L11 bodies 6
sketch "Sketch116" plane through (0, 0, 0) normal (0, 0, 1) x (1, 0, 0)
  line L0 (90, -75) -> (100, -75)
  line L1 (100, -75) -> (100, -85)
  line L2 (100, -85) -> (90, -85)
  line L3 (90, -85) -> (90, -75)
  line L4 (100, -75) -> (162.3, -75)
  line L5 (162.3, -75) -> (162.3, -85)
  line L6 (162.3, -85) -> (100, -85)
  line L7 (100, -85) -> (100, -75)
  line L8 (162.3, -75) -> (172.3, -75)
  line L9 (172.3, -75) -> (172.3, -85)
  line L10 (172.3, -85) -> (162.3, -85)
  line L11 (162.3, -85) -> (162.3, -75)
  line L12 (110, -85) -> (115, -85)
  line L13 (115, -85) -> (115, -90)
  line L14 (115, -90) -> (110, -90)
  line L15 (110, -90) -> (110, -85)
  line L16 (152.3, -85) -> (147.3, -85)
  line L17 (147.3, -85) -> (147.3, -90)
  line L18 (147.3, -90) -> (152.3, -90)
  line L19 (152.3, -90) -> (152.3, -85)
  line L20 (115, -90) -> (116, -90)
  line L21 (116, -90) -> (115, -85)
  line L22 (110, -90) -> (109, -90)
  line L23 (109, -90) -> (110, -85)
  line L24 (147.3, -90) -> (146.3, -90)
  line L25 (146.3, -90) -> (147.3, -85)
  line L26 (152.3, -90) -> (153.3, -90)
  line L27 (153.3, -90) -> (152.3, -85)
  dimension "d873" = 10
  dimension "d874" = 10
  dimension "d877" = 62.3
  dimension "d878" = 10
  dimension "d879" = 10
  dimension "d880" = 10
  dimension "d885" = 10
  dimension "d886" = 10
  dimension "d887" = 1
  dimension "d888" = 1
  dimension "d889" = 1
  dimension "d890" = 1
  dimension "d1013" = 5
  dimension "d1014" = 5
  dimension "d1015" = 5
  constraint horizontal L0
  constraint vertical L1
  constraint horizontal L2
  constraint vertical L3
  constraint horizontal L4
  constraint vertical L5
  constraint horizontal L6
  constraint vertical L7
  constraint horizontal L8
  constraint vertical L9
  constraint horizontal L10
  constraint vertical L11
  constraint horizontal L12
  constraint vertical L13
  constraint horizontal L14
  constraint vertical L15
  constraint coincident L6 L12.start
  constraint horizontal L16
  constraint vertical L17
  constraint horizontal L18
  constraint vertical L19
  constraint coincident L6 L16.start
  constraint perpendicular L13 L20
  constraint perpendicular L15 L22
  constraint perpendicular L19 L24
  constraint parallel L23 L25
  constraint perpendicular L19 L26
  measures "d873" distance of L0.start L0.end
  measures "d874" distance of L0.start L2.end
  measures "d877" distance of L0.end L4.end
  measures "d878" distance of L0.end L1.end
  measures "d879" distance of L4.end L8.end
  measures "d880" distance of L4.end L5.end
  measures "d885" distance of L1.end L15
  measures "d886" distance of L5.end L19
  measures "d887" distance of L13.end L20.end
  measures "d888" distance of L14.end L22.end
  measures "d889" distance of L17.end L24.end
  measures "d890" distance of L18.end L26.end
  measures "d1013" distance of L16.start L16.end
  measures "d1014" distance of L12.start L12.end
  measures "d1015" distance of L16.end L17.end
extrude "Extrude155" add sketch "Sketch116" against normal blind 5 separate body contours L0 L1 L2 L3 L7 | L5 L8 L9 L10 L11 makes body 7 at (93.3333, -78.3333, 0) makes body 8 at (165.6333, -78.3333, 0)
extrude "Extrude156" add sketch "Sketch116" along normal blind 3.5 contours L0 L1 L2 L3 L7 | L5 L8 L9 L10 L11 bodies 7 8
extrude "Extrude157" add sketch "Sketch116" along normal blind 50 contours L1 L4 L5 L6 L7 L11 L12 L16 | L6 L12 L13 L14 L15 | L15 L22 L23 | L13 L20 L21 | L6 L16 L17 L18 L19 | L19 L26 L27 | L17 L24 L25 bodies 7 8
sketch "Sketch117" plane through (0, 0, 3.5) normal (0, 0, 1) x (-1, 0, 0)
  line L0 (-90, 85) -> (-100, 85)
  line L1 (-100, 85) -> (-100, 75)
  line L2 (-100, 75) -> (-90, 75)
  line L3 (-90, 75) -> (-90, 85)
  circle A0 centre (-95, 80) radius 2.5
  dimension "d893" = 5
  measures "d893" diameter of A0
sketch "Sketch118" plane through (0, 0, 3.5) normal (0, 0, 1) x (-1, 0, 0)
  line L0 (-162.3, 85) -> (-172.3, 85)
  line L1 (-172.3, 85) -> (-172.3, 75)
  line L2 (-172.3, 75) -> (-162.3, 75)
  line L3 (-162.3, 75) -> (-162.3, 85)
  circle A0 centre (-167.3, 80) radius 2.5
  dimension "d894" = 5
  measures "d894" diameter of A0
extrude "Extrude158" cut sketch "Sketch118" sketch "Sketch117" against normal blind 10 contours A0 of sketch 2 contours A0 bodies 7
sketch "Sketch119" plane through (0, 0, 50) normal (0, 0, 1) x (-1, 0, 0)
  line L0 (-146.3, 90) -> (-153.3, 90)
  line L1 (-153.3, 90) -> (-152.3, 85)
  line L2 (-152.3, 85) -> (-162.3, 85)
  line L3 (-162.3, 85) -> (-162.3, 75)
  line L4 (-162.3, 75) -> (-100, 75)
  line L5 (-100, 75) -> (-100, 85)
  line L6 (-100, 85) -> (-110, 85)
  line L7 (-110, 85) -> (-109, 90)
  line L8 (-109, 90) -> (-116, 90)
  line L9 (-116, 90) -> (-115, 85)
  line L10 (-115, 85) -> (-147.3, 85)
  line L11 (-147.3, 85) -> (-146.3, 90)
  circle A0 centre (-105, 80) radius 2.5
  line L12 (-100, 85) -> (-100, 75)
  circle A1 centre (-157.3, 80) radius 2.5
  line L13 (-162.3, 75) -> (-162.3, 85)
  line L14 (-110, 85) -> (-152.3, 85)
  line L15 (-152.3, 85) -> (-152.3, 75)
  line L16 (-152.3, 75) -> (-110, 75)
  line L17 (-110, 75) -> (-110, 85)
  dimension "d897" = 5
  dimension "d898" = 5
  dimension "d899" = 5
  dimension "d900" = 5
  constraint horizontal L14
  constraint vertical L15
  constraint horizontal L16
  constraint vertical L17
  constraint coincident L4 L15.end
  constraint coincident L6.end L7.start
  measures "d897" diameter of A0
  measures "d898" distance of A0.centre L12
  measures "d899" diameter of A1
  measures "d900" distance of A1.centre L13
extrude "Extrude159" cut sketch "Sketch119" against normal blind 20 contours A0 | A1 bodies 7